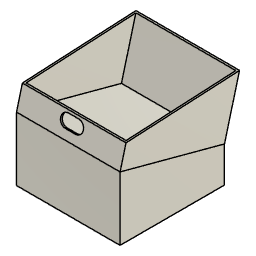
xbox-elite-s2-controller-holder v4 (Autodesk Fusion 360 design; units mm, degrees)
Autodesk Fusion 360 part; units mm, degrees
sketch "Sketch1" plane through (0, 0, 0) normal (0, 0, 1) x (1, 0, 0)
  line L0 (-95, 25) -> (-38, 25)
  line L1 (-38, 25) -> (-38, 84.5)
  line L2 (-38, 84.5) -> (-95, 84.5)
  line L3 (-95, 84.5) -> (-95, 25)
  dimension "d1" = 57
  dimension "d2" = 59.5
  constraint horizontal L0
  constraint vertical L1
  constraint horizontal L2
  constraint vertical L3
  measures "d1" distance of L0.start L0.end
  measures "d2" distance of L0.start L2.end
extrude "Extrude1" add sketch "Sketch1" along normal blind 32 makes body 1
shell "Shell1" thickness 1 removed faces 1 at (-76, 64.6667, 32) on bodies 1
draft "Draft1" angle -18 neutral plane through (-38, 84.5, 0) pull (0, 1, 0) 1 faces at (-94.6667, 64.3333, 32) on bodies 1
sketch "Sketch4" plane through (0, 25, 0) normal (0, -1, 0) x (1, 0, 0)
  line L0 (-95, 0) -> (-38, 0)
  line L1 (-38, 0) -> (-38, 12.6673)
  line L2 (-38, 12.6673) -> (-95, 12.6673)
  line L3 (-95, 12.6673) -> (-95, 0)
  line L4 (-63.6, 11.35) -> (-69.4, 11.35)
  arc A0 (-69.4, 11.35) -> (-69.4, 4.65) centre (-69.4, 8) ccw
  line L5 (-69.4, 4.65) -> (-63.6, 4.65)
  arc A1 (-63.6, 4.65) -> (-63.6, 11.35) centre (-63.6, 8) ccw
  line L6 (-60.25, 8) -> (-72.75, 8) construction
  dimension "d15" = 12.5
  dimension "d16" = 6.7
  constraint tangent L4 A0
  constraint tangent A0 L5
  constraint parallel L4 L5
  constraint tangent L5 A1
  constraint tangent L4 A1
  constraint midpoint A1 L6.start
  constraint midpoint A0 L6.end
  constraint horizontal L6
  measures "d15" distance of L6.start L6.end
  measures "d16" diameter of A0
extrude "Extrude4" cut sketch "Sketch4" against normal blind 1 contours L4 A0 L5 A1 bodies 1
sketch "Sketch6" plane through (0, 0, 0) normal (0, 0, 1) x (1, 0, 0)
  line L0 (-197, 85) -> (-140, 85)
  line L1 (-140, 85) -> (-140, 27.599)
  line L2 (-140, 27.599) -> (-197, 27.599)
  line L3 (-197, 27.599) -> (-197, 85)
  dimension "d19" = 57
  dimension "d20" = 57.401
  constraint horizontal L0
  constraint vertical L1
  constraint horizontal L2
  constraint vertical L3
  measures "d19" distance of L1.end L2.end
  measures "d20" distance of L0.start L2.end
extrude "Extrude5" add sketch "Sketch6" along normal blind 35 separate body makes body 2
move_body "Move1" bodies 1 to x (1, 0, 0) y (0, 0.965926, -0.258819) z (0, 0.258819, 0.965926) at (-102, 3.4519, 41.4705)
draft "Draft2" angle -15 neutral plane through (-140, 27.599, 0) pull (0, -1, 0) 1 faces at (-159, 65.8663, 35) on bodies 2
